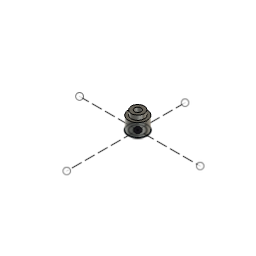
sphere2_disk_back v2 (Autodesk Fusion 360 design; units mm, degrees)
Autodesk Fusion 360 part; units mm, degrees
sketch "Skizze1" plane through (0, 0, 0) normal (0, 0, 1) x (1, 0, 0)
  line L0 (-31.5508, 0) -> (33.8224, 0) construction
  line L1 (0, 25.6192) -> (0, -38.4919) construction
  circle A0 centre (0, 0) radius 1.75
  circle A1 centre (0, 0) radius 3.5
  circle A2 centre (0, 0) radius 5
  dimension "d1" = 3.5
  dimension "d2" = 7
  dimension "d3" = 10
  constraint horizontal L0
  constraint coincident A0.centre L0
  constraint vertical L1
  constraint coincident A0.centre L1
  constraint coincident A0.centre A1.centre
  measures "d1" diameter of A0
  measures "d2" diameter of A1
  measures "d3" diameter of A2
extrude "Extrusion1" add sketch "Skizze1" along normal blind 7 contours A1 | A2
extrude "Extrusion2" add sketch "Skizze1" along normal blind 9.5 contours A1
ref_plane "Arbeitsebene1" through (0, 0, 3.5) normal (0, 0, 1) x (1, 0, 0)
sketch "Skizze2" plane through (0, 0, 3.5) normal (0, 0, 1) x (1, 0, 0)
  line L0 (-11, 0) -> (19, 0) construction
  line L1 (0, 16) -> (0, -23) construction
  line L2 (1.6743, -2.9) -> (3.3486, 0)
  line L3 (3.3486, 0) -> (1.6743, 2.9)
  line L4 (1.6743, 2.9) -> (-1.6743, 2.9)
  line L5 (-1.6743, 2.9) -> (-3.3486, 0)
  line L6 (-3.3486, 0) -> (-1.6743, -2.9)
  line L7 (-1.6743, -2.9) -> (1.6743, -2.9)
  dimension "d9" = 5.8
  constraint horizontal L0
  constraint coincident L0 origin
  constraint vertical L1
  constraint coincident L1 origin
  measures "d9" distance of L4 L7
extrude "Extrusion3" cut sketch "Skizze2" along normal mid plane 2.8
